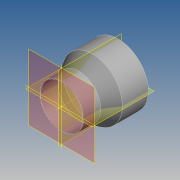
# Autodesk Inventor part: P011_Canon_AdaptVentilo
Saved by Autodesk Inventor 2020 (Build 240168000, 168)
## iProperties
Created: 2021-10-19
Part Number: P011_Canon_AdaptVentilo
Material: Générique
Document SubType Name: Modeling
Designer: gabri
Density: 1 g/cm^3
Appearance: Par défaut
Author: gabri
Autodesk Inventor part; units mm, degrees
sketch "Esquisse2" plane through (0, 0, 0) normal (0, 0, 1) x (1, 0, 0)
  line L0 (0, 43.3348) -> (0, -65.7143)
  line L1 (34, 65) -> (34, 35.1756)
  line L2 (34, 35.1756) -> (24.4, 20.1756)
  line L3 (24.4, 20.1756) -> (24.4, 0)
  line L4 (24.4, 0) -> (25, 0)
  line L5 (25, 0) -> (25, 20)
  line L6 (25, 20) -> (34.6, 35)
  line L7 (34.6, 35) -> (34.6, 65)
  line L8 (34.6, 65) -> (34, 65)
  line L9 (-6.92, 0) -> (41.52, 0) construction
  line L10 (0, 91.1429) -> (0, -91.8571) construction
  point P0 (0, 0)
  point P1 (24.7, 0)
  dimension "d1" = 68
  dimension "d2" = 0.6
  dimension "d3" = 0.6
  dimension "d4" = 0.6
  dimension "d5" = 20
  dimension "d6" = 15
  dimension "d7" = 30
  dimension "d8" = 34
  dimension "d11" = 25
  constraints: 18 end point, 4 parallel, 3 perpendicular, 2 vertical, 1 midpoint, 1 point on line
  measures "d1" diameter of L1 L0
  measures "d2" distance of L3.end L4.end
  measures "d3" distance of L7.end L1.start
  measures "d4" distance between parallel lines of L6 L2
  measures "d5" distance of L4.end L5.end
  measures "d6" vertical distance of L6.end L5.end
  measures "d7" distance of L7.end L6.end
  measures "d8" distance between parallel lines of L10 L1
  measures "d11" distance between parallel lines of L10 L5
revolve "Révolution1" add sketch "Esquisse2" angle 360 about axis through (0, 43.3348, 0) along (0, -1, 0)
